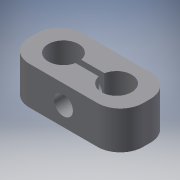
# Autodesk Inventor part: crank web
Saved by Autodesk Inventor 2016 (Build 200138000, 138)
## iProperties
Created: 2017-06-14
Part Number: crank web
Material: Generic
Document SubType Name: Modeling
Designer: RMcComber
Density: 1 g/cm^3
Appearance: Default
Author: RMcComber
Autodesk Inventor part; units mm, degrees
ref_plane "YZ Plane" through (0, 0, 0) normal (1, 0, 0) x (0, 1, 0)
ref_plane "XZ Plane" through (0, 0, 0) normal (0, 1, 0) x (-1, 0, 0)
ref_plane "XY Plane" through (0, 0, 0) normal (0, 0, 1) x (1, 0, 0)
sketch "Sketch1" plane through (0, 0, 0) normal (0, 0, 1) x (1, 0, 0)
  line L0 (0, 0) -> (-14, 0) construction
  circle A0 centre (-14, 0) radius 4
  circle A1 centre (0, 0) radius 4
  line L1 (8, -7) -> (-22, -7)
  line L2 (-22, -7) -> (-22, 7)
  line L3 (-22, 7) -> (8, 7)
  line L4 (8, 7) -> (8, -7)
  line L5 (8, -7) -> (-22, 7) construction
  line L6 (-22, -7) -> (8, 7) construction
  point P0 (-7, 0)
  dimension "d0" = 8
  dimension "d1" = 14
  dimension "d2" = 8
  dimension "d3" = 14
  dimension "d13" = 30
  constraints: 14 end point, 3 midpoint, 2 centre point, 2 coincident, 2 horizontal, 2 parallel, 1 equal radius, 1 perpendicular
  measures "d0" diameter of A0
  measures "d1" distance of L0.start L0.end
  measures "d2" distance from line of L0.end L2
  measures "d3" distance of L3.end L1.start
  measures "d13" distance of L1.start L1.end
extrude "Extrusion1" add sketch "Sketch1" along normal blind 10
sketch "Sketch2" plane through (-22, 7, 0) normal (0, 1, 0) x (1, 0, 0)
  line L0 (0, 0) -> (30, 0) projected
  line L1 (30, -10) -> (0, -10) projected
  line L2 (15, 0) -> (15, -10) construction
  circle A0 centre (15, -5) radius 2.5
  point P0 (22, 0)
  dimension "d6" = 5
  constraints: 3 midpoint, 2 end point, 1 centre point
  measures "d6" diameter of A0
extrude "Extrusion2" cut sketch "Sketch2" against normal through all
fillet "Fillet1" radius 6 4 edges at (8, 7, 5) (-22, 7, 5) (-22, -7, 5) (8, -7, 5)
sketch "Sketch3" plane through (0, 0, 10) normal (0, 0, 1) x (1, 0, 0)
  line L0 (-16, -7) -> (2, -7) projected
  circle A0 centre (0, 0) radius 4 projected
  circle A1 centre (-14, 0) radius 4 projected
  line L1 (-14, 0) -> (0, 0) construction
  line L2 (0, -0.75) -> (-14, -0.75)
  line L3 (-14, -0.75) -> (-14, 0.75)
  line L4 (-14, 0.75) -> (0, 0.75)
  line L5 (0, 0.75) -> (0, -0.75)
  line L6 (0, -0.75) -> (-14, 0.75) construction
  line L7 (-14, -0.75) -> (0, 0.75) construction
  point P0 (-7, 0)
  dimension "d10" = 1.5
  constraints: 14 end point, 4 midpoint, 3 parallel, 1 horizontal, 1 perpendicular
  measures "d10" distance of L2.end L3.end
extrude "Extrusion3" cut sketch "Sketch3" against normal through all contours L4 L5 L2 A0 | A0 L2 A1 L4 | A1 L2 L3 L4 picked at (-1.3307, -0.0838) picked at (-12.6667, 0)
body "Solid1"
